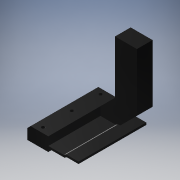
# Autodesk Inventor part: GA04
Saved by Autodesk Inventor 2017 (Build 210142000, 142)
## iProperties
Created: 2018-10-24
Part Number: GA04
Material: ABS Plastic
Document SubType Name: Modeling
Designer: Dell
Density: 1.06 g/cm^3
Appearance: Smooth - Black
Author: Dell
Autodesk Inventor part; units mm, degrees
ref_plane "YZ Plane" through (0, 0, 0) normal (1, 0, 0) x (0, 1, 0)
ref_plane "XZ Plane" through (0, 0, 0) normal (0, 1, 0) x (-1, 0, 0)
ref_plane "XY Plane" through (0, 0, 0) normal (0, 0, 1) x (1, 0, 0)
sketch "Sketch9" plane through (0, 0, 0) normal (0, 0, 1) x (1, 0, 0)
  line L0 (0, 0) -> (0, 55) construction
  circle A0 centre (0, 55) radius 1.5
  circle A1 centre (0, 0) radius 1.5
  circle A2 centre (0, 27.5) radius 1.5
  line L1 (-10, 60) -> (10, 60)
  line L2 (10, 60) -> (10, -5)
  line L3 (10, -5) -> (-10, -5)
  line L4 (-10, -5) -> (-10, 60)
  point P0 (-10, 27.5)
  point P1 (0, 60)
  dimension "d35" = 55
  dimension "d36" = 3
  dimension "d37" = 3
  dimension "d38" = 3
  dimension "d39" = 5
  dimension "d40" = 10
  constraints: 10 end point, 3 centre point, 3 midpoint, 2 coincident, 2 parallel, 1 horizontal, 1 horizontal alignment, 1 perpendicular, 1 vertical, 1 vertical alignment
  measures "d35" distance of L0.start L0.end
  measures "d36" diameter of A0
  measures "d37" diameter of A1
  measures "d38" diameter of A2
  measures "d39" distance from line of L1 L0.end
  measures "d40" distance between parallel lines of L4 L0
extrude "Extrusion9" add sketch "Sketch9" along normal blind 10
sketch "Sketch11" plane through (10, -5, 0) normal (1, 0, 0) x (0, 0, -1)
  line L0 (0, 65) -> (-10, 65) projected
  line L1 (0, 65) -> (-75, 65)
  line L2 (-75, 65) -> (-75, 50)
  line L3 (-75, 50) -> (0, 50)
  line L4 (0, 50) -> (0, 65)
  point P0 (0, 5)
  dimension "d43" = 15
  dimension "d44" = 75
  constraints: 8 end point, 2 parallel, 1 horizontal, 1 perpendicular
  measures "d43" distance between parallel lines of L3 L1
  measures "d44" distance of L0.start L1.end
extrude "Extrusion10" add sketch "Sketch11" along normal blind 35
sketch "Sketch12" plane through (-10, 60, 10) normal (0, 1, 0) x (1, 0, 0)
  line L0 (20, -65) -> (20, 0) projected
  line L1 (20, -65) -> (34, -65)
  line L2 (34, -65) -> (34, 0)
  line L3 (34, 0) -> (20, 0)
  line L4 (20, 0) -> (20, -65)
  point P0 (10, 10)
  dimension "d47" = 14
  constraints: 8 end point, 2 parallel, 1 horizontal, 1 perpendicular, 1 point on line
  measures "d47" distance between parallel lines of L2 L0
extrude "Extrusion11" cut sketch "Sketch12" against normal through all
chamfer "Chamfer6" distance 14 angle 45 1 edges at (24, 52.5, 10)
sketch "Sketch14" plane through (10, 45, 0) normal (0, -1, 0) x (1, 0, 0)
  line L0 (0, 10) -> (14, 24) projected
  line L1 (15.4558, 0) -> (35, 19.5442)
  line L2 (35, 75) -> (35, 0) projected
  line L3 (0, 0) -> (35, 0) projected
  line L4 (15.4558, 0) -> (35, 0)
  line L5 (35, 19.5442) -> (35, 0)
  point P0 (-10, 0)
  dimension "d73" = 18
  constraints: 6 end point, 2 point on line, 1 horizontal, 1 parallel, 1 perpendicular
  measures "d73" distance between parallel lines of L0 L1
extrude "Extrusion13" cut sketch "Sketch14" against normal through all
sketch "Sketch15" plane through (0, 0, 0) normal (0, 0, -1) x (-1, 0, 0)
  line L0 (-25.4558, 60) -> (-25.4558, 45) projected
  line L1 (-10, 45) -> (-25.4558, 45) projected
  line L2 (-10, 45) -> (-10, -5) projected
  line L3 (-10, -5) -> (10, -5) projected
  line L4 (10, -5) -> (10, 60) projected
  line L5 (10, 60) -> (-25.4558, 60) projected
  circle A0 centre (0, 55) radius 1.5 projected
  circle A1 centre (0, 0) radius 1.5 projected
  circle A2 centre (0, 27.5) radius 1.5 projected
  line L6 (-10, -5) -> (10, -5) projected
  line L7 (10, 60) -> (-10, 60) projected
  line L8 (-10, -5) -> (-10, 60)
  line L9 (-10, 60) -> (10, 60)
  constraints: 4 end point, 1 collinear, 1 perpendicular
extrude "Extrusion14" add sketch "Sketch15" along normal blind 3 contours L5 L4 L3 L2 L8
chamfer "Chamfer8" distance 3 angle 45 1 edges at (-10, 27.5, 10)
sketch "Sketch17" plane through (-10, -5, -3) normal (0, -1, 0) x (1, 0, 0)
  line L0 (20, 3) -> (20, 13) projected
  line L1 (20, 3) -> (35.4558, 3) projected
  line L2 (20, 3) -> (35.4558, 3)
  line L3 (35.4558, 3) -> (37.5981, 4.5)
  line L4 (37.5981, 4.5) -> (49, 4.5)
  line L5 (49, 6.5) -> (36.9675, 6.5)
  line L6 (36.9675, 6.5) -> (34.8252, 5)
  line L7 (34.8252, 5) -> (20, 5)
  line L8 (20, 3) -> (20, 5)
  line L9 (49, 6.5) -> (49, 4.5)
  point P0 (10, 3)
  point P1 (55, 22.5442)
  dimension "d83" = 215
  dimension "d84" = 2
  dimension "d88" = 1.5
  dimension "d89" = 6
  constraints: 16 end point, 3 parallel, 2 collinear, 2 other
  measures "d84" distance between parallel lines of L3 L6
  measures "d88" distance between parallel lines of L1 L4
  measures "d89" horizontal distance of point (55, 22.544) L4.end
extrude "Extrusion16" add sketch "Sketch17" against normal blind 65
equation "\"Module\" = 2"
equation "\"PressureAngle\" = 20deg"
equation "\"UnitProfileClearance\" = 0.25"
equation "\"UnitRoundRadius\" = 0.35"
equation "\"HeadDiameter\" = 42"
equation "\"RootDiameter\" = 33"
equation "\"BaseDiameter\" = 35.70832"
equation "\"PitchDiameter\" = 38"
equation "\"HelixAngle\" = 0"
equation "\"UnitCorrection\" = 0"
equation "\"UnitAddendumModification\" = 0"
equation "\"CircularPitch\" = 6.283185"
equation "\"UnitBacklashShift\" = 0"
equation "\"TotalToolShift\" = 0"
equation "\"IsInternal\" = 0"
body "Solid3"
